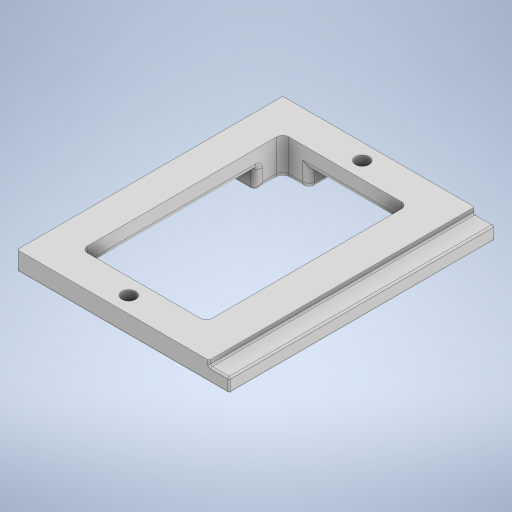
# Autodesk Inventor part: BacklightCaseMountUnder
Saved by Autodesk Inventor 2023 (Build 270158000, 158)
## iProperties
Created: 2026-02-11
Part Number: BacklightCaseMountUnder
Material: Generic
Document SubType Name: Modeling
Designer: DanAr
Density: 1 g/cm^3
Appearance: Default
Author: DanAr
Autodesk Inventor part; units mm, degrees
ref_plane "YZ Plane" through (0, 0, 0) normal (1, 0, 0) x (0, 1, 0)
ref_plane "XZ Plane" through (0, 0, 0) normal (0, 1, 0) x (-1, 0, 0)
ref_plane "XY Plane" through (0, 0, 0) normal (0, 0, 1) x (1, 0, 0)
sketch "Sketch1" plane through (0, 0, 0) normal (0, 1, 0) x (-1, 0, 0)
  line L0 (0, 0) -> (47.7, 0)
  line L1 (47.7, 0) -> (47.7, -66)
  line L2 (47.7, -66) -> (0, -66)
  line L3 (0, -66) -> (0, 0)
  dimension "d0" = 66
  dimension "d1" = 47.7
  constraints: 8 end point, 2 parallel, 1 horizontal, 1 perpendicular
  measures "d0" distance of L0.end L1.end
  measures "d1" distance of L1.end L2.end
extrude "Extrusion1" add sketch "Sketch1" along normal blind 4.7
sketch "Sketch2" plane through (0, 0, 0) normal (0, -1, 0) x (1, 0, 0)
  line L0 (0, -66) -> (-47.7, -66) projected
  line L1 (-47.7, -66) -> (-33.2, -66)
  line L2 (-33.2, -66) -> (-33.2, -51.5)
  line L3 (-33.2, -51.5) -> (-47.7, -51.5)
  line L4 (-47.7, -51.5) -> (-47.7, -66)
  point P0 (0, 0)
  dimension "d4" = 14.5
  dimension "d5" = 14.5
  constraints: 8 end point, 2 parallel, 1 horizontal, 1 perpendicular
  measures "d4" distance of L2.end L3.end
  measures "d5" distance of L1.end L2.end
extrude "Extrusion2" add sketch "Sketch2" along normal blind 4.7
fillet "Fillet1" radius 0.2 1 edges at (-40.45, 0, -51.5)
fillet "Fillet2" radius 0.4 4 edges at (-23.85, 0, 0) (-40.45, -4.7, -51.5) (-40.45, -4.7, -66) (-16.6, 0, -66)
sketch "Sketch3" plane through (0, 4.7, 0) normal (1, 0, 0) x (0, 0, -1)
  line L0 (0, 0) -> (66, 0) projected
  line L1 (66, -4.3) -> (66, 0) projected
  line L2 (0, 0) -> (66, 0)
  line L3 (66, 0) -> (66, -1.3)
  line L4 (66, -1.3) -> (0, -1.3)
  line L5 (0, -1.3) -> (0, 0)
  line L6 (66, -1.3) -> (0, -1.3)
  line L7 (0, -1.3) -> (0, -4.7)
  line L8 (0, -4.7) -> (66, -4.7)
  line L9 (66, -4.7) -> (66, -1.3)
  point P0 (0, -1.3)
  dimension "d10" = 1.3
  constraints: 16 end point, 4 parallel, 2 horizontal, 2 perpendicular, 1 point on line
  measures "d10" distance between parallel lines of L0 L4
extrude "Extrusion3" add sketch "Sketch3" along normal blind 5 contours L4 L1 L9 L8 L7
fillet "Fillet3" radius 0.4 2 edges at (2.5, 0, 0) (2.5, 0, -66)
sketch "Sketch4" plane through (0, 4.7, 0) normal (0, 1, 0) x (1, 0, 0)
  line L0 (-71.45, 4) -> (-23.95, 4)
  line L1 (-23.95, 4) -> (-23.95, 62)
  line L2 (-23.95, 62) -> (-71.45, 62)
  line L3 (-71.45, 62) -> (-71.45, 4)
  line L4 (-47.7, 66) -> (-47.7, 0) projected
  line L5 (-71.45, 4) -> (-23.95, 62) construction
  line L6 (-23.95, 4) -> (-71.45, 62) construction
  circle A0 centre (-23.95, 62) radius 1.7
  circle A1 centre (-23.95, 4) radius 1.7
  line L7 (-23.95, 62) -> (-24.2, 62)
  line L8 (-24.2, 62) -> (-24.2, 4)
  line L9 (-24.2, 4) -> (-23.95, 4)
  line L10 (-23.95, 4) -> (-23.95, 62)
  line L11 (-8.7, 58) -> (-39.7, 58)
  line L12 (-39.7, 58) -> (-39.7, 8)
  line L13 (-39.7, 8) -> (-8.7, 8)
  line L14 (-8.7, 8) -> (-8.7, 58)
  line L15 (-8.7, 58) -> (-39.7, 8) construction
  line L16 (-39.7, 58) -> (-8.7, 8) construction
  point P0 (0, 0)
  point P1 (-47.7, 33)
  point P2 (-24.2, 33)
  dimension "d14" = 58
  dimension "d15" = 47.5
  dimension "d16" = 3.4
  dimension "d17" = 0.25
  dimension "d18" = 31
  dimension "d19" = 50
  constraints: 32 end point, 6 midpoint, 6 parallel, 3 horizontal, 3 perpendicular, 2 centre point, 2 coincident, 1 point on line
  measures "d14" distance of L2.end L0.start
  measures "d15" distance of L1.end L2.end
  measures "d16" diameter of A0
  measures "d17" distance between parallel lines of L8 L1
  measures "d18" distance of L11.start L11.end
  measures "d19" distance of L11.end L12.end
extrude "Extrusion4" cut sketch "Sketch4" against normal blind 10 contours L8 A1 L1 L0 | L0 L1 A1 | L0 A1 L8 | L13 L12 L11 L8 | L8 L11 L1 L13 | L1 L11 L14 L13 | A0 L1 L2 | L2 L8 A0 | L8 L2 L1 A0
chamfer "Chamfer1" distance 0.3 angle 45 2 edges at (-25.65, 0, -4) (-25.65, 0, -62)
fillet "Fillet4" radius 1.5 4 edges at (-39.7, 0, -58) (-8.7, 2.35, -58) (-39.7, 2.35, -8) (-8.7, 2.35, -8)
fillet "Fillet5" radius 1.5 17 edges at (-39.7, 0, -30.4) (-39.2607, 0, -8.4393) (-24.2, 0, -8) (-9.1393, 0, -8.4393) (-8.7, 0, -33) (-9.1393, 0, -57.5607) (-21.7, 0, -58) (-39.7, -0.0586, -51.4414) (-39.7, -2.25, -51.5) (-39.7, -4.5828, -51.6172) (-39.7, -4.7, -54.2) (-39.2607, -4.7, -57.5607) (-35.7, -4.7, -58) (-33.2, -2.35, -58) (-33.2, -4.5828, -65.8828) (-33.2, -1.95, -66) (-33.2, -4.7, -61.8)
fillet "Fillet6" radius 0.4 24 edges at (5, 3.4, -33) (5, 0.1171, -65.8829) (5, 0, -33) (5, 0.1171, -0.1171) (5, 1.8999, 0) (5, 1.9, -66) (2.5, 3.4, -66) (2.5, 3.4, 0) (0, 4.05, -66) (0, 4.05, 0) (0, 3.4, -33) (-33.3253, 0, -65.1001) (-34.1543, 0.1323, -65.8972) (-33.6393, 0.4393, -58.4393) (-33.2, 0, -62) (-47.7, 0.1172, -0.1172) (-47.7, 2.55, 0) (-47.7, -0.0586, -51.4414) (-47.7, -2.25, -51.5) (-47.7, -4.5828, -51.6172) (-47.7, -4.7, -58.75) (-47.7, -4.5828, -65.8828) (-47.7, 0.2, -66) (-47.7, 0, -25.85)
body "Solid1"
